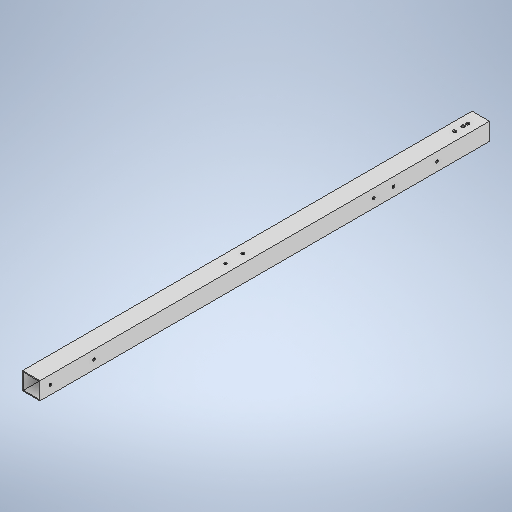
# Autodesk Inventor part: kaku_2020_465
Saved by Autodesk Inventor 2025.1 (Build 291241000, 241)
## iProperties
Created: 2024-10-08
Part Number: kaku_2020_465
Material: 一般
Document SubType Name: Modeling
Designer: yuki0520
Density: 1 g/cm^3
Appearance: 既定
Author: yuki0520
Autodesk Inventor part; units mm, degrees
ref_plane "YZ Plane" through (0, 0, 0) normal (1, 0, 0) x (0, 1, 0)
ref_plane "XZ Plane" through (0, 0, 0) normal (0, 1, 0) x (-1, 0, 0)
ref_plane "XY Plane" through (0, 0, 0) normal (0, 0, 1) x (1, 0, 0)
sketch "スケッチ1" plane through (0, 0, 0) normal (0, 0, 1) x (1, 0, 0)
  line L0 (10, -10) -> (-10, -10)
  line L1 (-10, -10) -> (-10, 10)
  line L2 (-10, 10) -> (10, 10)
  line L3 (10, 10) -> (10, -10)
  line L4 (10, -10) -> (-10, 10) construction
  line L5 (-10, -10) -> (10, 10) construction
  line L6 (9, 9) -> (-9, 9)
  line L7 (-9, 9) -> (-9, -9)
  line L8 (-9, -9) -> (9, -9)
  line L9 (9, -9) -> (9, 9)
  point P0 (0, 0)
  dimension "d0" = 20
  dimension "d1" = 20
  dimension "d2" = 1
  constraints: 20 end point, 4 parallel, 2 midpoint, 2 perpendicular, 1 horizontal, 3 other
  measures "d0" distance of L1.end L2.end
  measures "d1" distance of L0.end L1.end
  measures "d2" distance between parallel lines of L2 L6
extrude "押し出し1" add sketch "スケッチ1" along normal blind 465
sketch "スケッチ2" plane through (10, -10, 0) normal (1, 0, 0) x (0, 0, -1)
  line L0 (0, 10) -> (-465, 10)
  line L1 (-465, 0) -> (-465, 20) projected
  line L2 (0, 0) -> (0, 20) projected
  point P0 (-403, 10)
  point P1 (-60, 10)
  point P2 (-10, 10)
  point P3 (-453, 10)
  point P4 (-82.5, 10)
  point P5 (-232.5, 10)
  dimension "d5" = 343
  dimension "d6" = 50
  dimension "d7" = 10
  dimension "d15" = 50
  dimension "d17" = 465
  dimension "d28" = 150
  constraints: 5 point on line, 2 end point, 2 midpoint, 1 horizontal
  measures "d5" distance of point (-60, 10) point (-403, 10)
  measures "d6" distance of point (-60, 10) point (-10, 10)
  measures "d7" distance from line of L2 point (-10, 10)
  measures "d15" distance of point (-453, 10) point (-403, 10)
  measures "d17" distance between parallel lines of L2 L1
  measures "d28" distance of point (-232.5, 10) point (-82.5, 10)
hole "穴1" at (10, 0, 403) at (10, 0, 60) at (10, 0, 10) at (10, 0, 453) at (10, 0, 82.5) direction (-1, 0, 0) diameter 3.3 end through all
sketch "スケッチ3" plane through (-10, 10, 0) normal (0, 1, 0) x (1, 0, 0)
  line L0 (10, 0) -> (10, -465)
  line L1 (20, -465) -> (0, -465) projected
  point P0 (10, -242.5)
  point P1 (10, -222.5)
  point P2 (10, -232.5)
  dimension "d19" = 20
  dimension "d20" = 10
  constraints: 2 end point, 2 midpoint, 2 point on line
  measures "d19" distance of point (10, -242.5) point (10, -222.5)
  measures "d20" distance of point (10, -232.5) point (10, -242.5)
hole "穴2" at (0, 10, 242.5) at (0, 10, 222.5) direction (0, -1, 0) diameter 3.3 end through all
sketch "スケッチ6" plane through (0, 0, 0) normal (0, 0, -1) x (-1, 0, 0)
  line L0 (-10, 10) -> (10, 10) projected
  line L1 (-10, -10) -> (-10, 10) projected
  line L2 (10, -10) -> (-10, -10) projected
  line L3 (10, 10) -> (10, -10) projected
  line L4 (-9, 9) -> (-9, -9) projected
  line L5 (9, 9) -> (-9, 9) projected
  line L6 (9, -9) -> (9, 9) projected
  line L7 (-9, -9) -> (9, -9) projected
  point P0 (0, 0)
extrude "押し出し4" add sketch "スケッチ6" along normal blind 50
sketch "スケッチ7" plane through (-10, 10, 465) normal (0, 1, 0) x (1, 0, 0)
  line L0 (10, 465) -> (10, 515)
  line L1 (1, 515) -> (19, 515) projected
  point P0 (10, 500)
  point P1 (10, 485)
  point P2 (10, 495)
  dimension "d44" = 35
  dimension "d52" = 10
  dimension "d53" = 5
  constraints: 3 point on line, 2 end point, 1 midpoint
  measures "d44" distance of L0.start point (10, 500)
  measures "d52" distance of point (10, 495) point (10, 485)
  measures "d53" distance of point (10, 500) point (10, 495)
hole "穴3" at (0, 10, -30) at (0, 10, -20) at (0, 10, -35) direction (0, -1, 0) diameter 4 end through all
